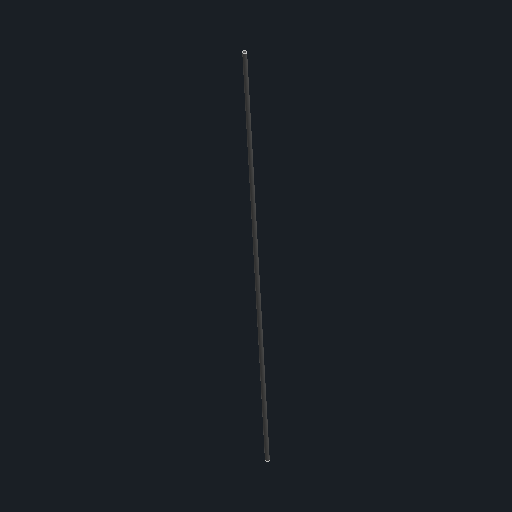
# Autodesk Inventor part: steering_rod
Saved by Autodesk Inventor 2024 (Build 280153000, 153)
## iProperties
Created: 2022-03-30
Part Number: steering_rod
Material: Generic
Document SubType Name: Modeling
Designer: kardo
Density: 1 g/cm^3
Appearance: Dark Plastic
Mass: 0.682366 g
Surface Area: 13.7101 cm^2
Volume: 0.682366 cm^3
Author: kardo
Autodesk Inventor part; units mm, degrees
ref_plane "YZ Plane" through (0, 0, 0) normal (1, 0, 0) x (0, 1, 0)
ref_plane "XZ Plane" through (0, 0, 0) normal (0, 1, 0) x (-1, 0, 0)
ref_plane "XY Plane" through (0, 0, 0) normal (0, 0, 1) x (1, 0, 0)
derived "stencil_frame.ipt"
sketch3d "sk_servo_rod"
ref_plane "Work Plane1" through (-9.6, -178.883, 43.7206) normal (-0.0340694, -0.9949963, -0.0939236) x (0.9994143, -0.0342207, 0)
sketch "Sketch1" plane through (-9.6, -178.883, 43.7206) normal (-0.0340694, -0.9949963, -0.0939236) x (0.9994143, -0.0342207, 0)
  circle A0 centre (0, 0) radius 1
  point P0 (3.4729, -60.3496)
  point P1 (0, 0)
  dimension "d1" = 2
  constraints: 1 centre point, 1 coincident
  measures "d1" diameter of A0
extrude "Extrusion1" add sketch "Sketch1" along normal up to surface (217.2038 mm away)
body "Solid1"
